Autodesk Inventor part; units mm, degrees
(part 3 of 3)
  spline S581 degree 2 poles (9.4337, -3.0832) (9.3792, -3.0832) (9.2544, -3.1501) (9.1886, -3.2137) knots 0 0 0 1 2 2 2
  spline S582 degree 2 poles (9.1886, -3.2137) (9.1898, -3.2296) (9.192, -3.2738) (9.192, -3.3033) knots 0 0 0 1 2 2 2
  line L532 (9.192, -3.3033) -> (9.192, -3.9954)
  line L533 (9.192, -3.9954) -> (9.0151, -3.9954)
  line L534 (9.0151, -3.9954) -> (9.0151, -3.3873)
  spline S583 degree 2 poles (9.0151, -3.3873) (9.0151, -3.3146) (9.0037, -3.191) (8.9856, -3.1569) knots 0 0 0 1 2 2 2
  spline S584 degree 2 poles (8.9856, -3.1569) (8.9674, -3.1195) (8.8982, -3.0832) (8.8381, -3.0832) knots 0 0 0 1 2 2 2
  spline S585 degree 2 poles (8.8381, -3.0832) (8.7813, -3.0832) (8.6554, -3.1547) (8.5964, -3.2103) knots 0 0 0 1 2 2 2
  line L535 (8.5964, -3.2103) -> (8.5964, -3.9954)
  line L536 (8.5964, -3.9954) -> (8.4194, -3.9954)
  line L537 (8.4194, -3.9954) -> (8.4194, -2.9448)
  line L538 (8.4194, -2.9448) -> (8.5964, -2.9448)
  line L539 (8.5964, -2.9448) -> (8.5964, -3.0605)
  spline S586 degree 2 poles (8.5964, -3.0605) (8.6656, -2.9913) (8.8018, -2.9153) (8.8835, -2.9153) knots 0 0 0 1 2 2 2
  spline S587 degree 2 poles (8.8835, -2.9153) (8.9765, -2.9153) (9.1206, -3.0004) (9.158, -3.0968) knots 0 0 0 1 2 2 2
  spline S588 degree 2 poles (9.158, -3.0968) (9.2386, -3.0072) (9.3906, -2.9153) (9.4791, -2.9153) knots 0 0 0 1 2 2 2
  spline S589 degree 2 poles (9.4791, -2.9153) (9.5471, -2.9153) (9.6583, -2.9573) (9.6992, -3.0049) knots 0 0 0 1 2 2 2
  spline S590 degree 2 poles (9.6992, -3.0049) (9.7412, -3.0526) (9.7877, -3.1955) (9.7877, -3.3033) knots 0 0 0 1 2 2 2
  line L540 (9.7877, -3.3033) -> (9.7877, -3.9954)
  line L541 (9.7877, -3.9954) -> (9.6107, -3.9954)
  line L542 (11.6188, -2.5954) -> (11.2671, -3.9954)
  line L543 (11.2671, -3.9954) -> (11.0583, -3.9954)
  line L544 (11.0583, -3.9954) -> (10.7736, -2.8336)
  line L545 (10.7736, -2.8336) -> (10.4967, -3.9954)
  line L546 (10.4967, -3.9954) -> (10.2903, -3.9954)
  line L547 (10.2903, -3.9954) -> (9.9329, -2.5954)
  line L548 (9.9329, -2.5954) -> (10.1246, -2.5954)
  line L549 (10.1246, -2.5954) -> (10.406, -3.756)
  line L550 (10.406, -3.756) -> (10.6851, -2.5954)
  line L551 (10.6851, -2.5954) -> (10.8745, -2.5954)
  line L552 (10.8745, -2.5954) -> (11.1559, -3.7696)
  line L553 (11.1559, -3.7696) -> (11.4361, -2.5954)
  line L554 (11.4361, -2.5954) -> (11.6188, -2.5954)
  point P0 (0, 0)
  point P1 (17.127, 0)
  constraints: 1 midpoint, 1 point on line, 2 other
extrude "Extrusion3" cut sketch "Sketch3" against normal blind 0.1 contours S211 S212 L234 L235 S213 S214 L5 | L5 S214 S215 S216 S222 S223 S224 S218 S219 S220 S207 S208 S209 S210 S211 | L5 S220 S221 S222 S216 S217 S206 S207 | S0 S1 L10 L11 L12 S2 S3 | L16 L17 L18 L19 L20 L21 | L22 L23 L24 L25 L26 L27 L28 L29 | L30 L31 S8 S9 S10 L32 L33 L34 L35 L36 S11 S12 L37 | S13 S14 S15 S16 | L38 S21 S22 L39 L40 L41 L42 L43 S23 S24 L44 | L45 L46 L47 L48 L49 L50 | S25 S26 S27 S28 S29 S30 L51 S31 S32 S33 L52 L53 S34 S35 S36 L54 L55 L56 | S41 S42 L58 L59 L60 L61 L62 S43 S44 | S49 L64 L65 S50 S51 S52 S53 S54 S55 S56 S57 S58 L66 L67 S59 S60 S61 S62 S63 S64 S65 | L68 L69 L70 L71 L72 L73 | S66 S67 L74 L75 L76 L77 L78 S68 S69 | L82 L83 L84 L85 L86 L87 L88 L89 L90 L91 L92 L93 L94 | L95 L96 L97 L98 | S74 S75 S76 S77 S78 S79 S80 L99 L100 S81 S82 S83 S84 S85 | S93 S94 L101 L102 S95 S96 S97 S98 L103 S99 S100 S101 S102 S103 L104 L105 S104 S105 S106 S107 S108 L106 L107 L108 S109 S110 S111 | S112 S113 S114 L109 L110 S115 S116 S117 S118 S119 S120 S121 L111 L112 L113 L114 L115 S122 S123 S124 | L116 L117 L118 L119 | S125 L120 L121 S126 S127 S128 S129 S130 S131 S132 S133 L122 L123 S134 S135 S136 S137 S138 S139 S140 | L124 L125 L126 L127 L128 L129 L130 L131 L132 L133 L134 L135 L136 | L137 L138 L139 L140 L141 L142 L143 L144 | S141 L148 L149 S142 S143 S144 S145 S146 S147 S148 S149 L150 L151 S150 S151 S152 S153 S154 S155 S156 | L152 L153 L154 L155 | L156 L157 L158 L159 L160 L161 L162 L163 L164 L165 | L166 L167 L168 L169 | L170 L171 L172 L173 | L174 L175 L176 L177 L178 L179 S157 L180 L181 L182 L183 | S158 S159 S160 S161 S162 S163 S164 L184 L185 S165 S166 S167 S168 S169 | L186 L187 L188 L189 L190 L191 S177 L192 L193 L194 L195 | L196 L197 L198 L199 L200 L201 S178 L202 L203 L204 L205 | L206 L207 L208 L209 L210 L211 S179 L212 L213 L214 L215 | S180 S181 S182 L216 L217 S183 S184 S185 S186 S187 S188 S189 L218 L219 L220 L221 L222 S190 S191 S192 | L223 L224 L225 L226 | S193 S194 S195 L227 L228 S196 S197 S198 S199 S200 S201 S202 L229 L230 L231 L232 L233 S203 S204 S205 | S225 S226 S227 S228 S229 S230 L236 L237 S231 S232 S233 S234 S235 S236 S237 S238 L238 L239 S239 S240 | S241 S242 S243 S244 L240 L241 S245 S246 S247 L242 L243 S248 S249 | L245 L246 S254 S255 S256 L247 L248 L249 L250 L251 S257 S258 L252 | S259 L253 L254 L255 L256 L257 L258 L259 L260 L261 L262 L263 S260 S261 S262 L264 L265 S263 | S264 S265 S266 S267 L266 L267 S268 S269 S270 L268 L269 S271 S272 | L271 S277 S278 L272 L273 L274 L275 L276 S279 S280 L277 | L278 L279 L280 L281 L282 L283 L284 L285 L286 L287 L288 L289 L290 | S281 S282 S283 S284 S285 S286 L291 S287 S288 S289 L292 L293 S290 S291 S292 L294 L295 L296 | L298 L299 L300 L301 L302 L303 L304 | S297 S298 S299 S300 L305 L306 S301 S302 S303 L307 L308 S304 S305 | L310 L311 L312 L313 | S310 S311 S312 S313 L314 L315 S314 S315 S316 L316 L317 S317 S318 | L319 L320 S323 S324 S325 L321 L322 L323 L324 L325 S326 S327 L326 | S328 S329 S330 S331 L327 S332 S333 S334 S335 S336 L328 L329 L330 S337 S338 L331 L332 | S343 L334 L335 L336 L337 L338 L339 L340 L341 L342 L343 L344 S344 S345 S346 L345 L346 S347 | L347 L348 S348 S349 S350 L349 L350 L351 L352 L353 S351 S352 L354 | L355 L356 L357 L358 | L359 L360 L361 L362 | S353 S354 S355 S356 S357 S358 S359 L363 L364 S360 S361 S362 S363 S364 | S372 S373 L365 L366 S374 S375 S376 S377 L367 S378 S379 S380 S381 S382 L368 L369 S383 S384 S385 S386 S387 L370 L371 L372 S388 S389 S390 | S391 S392 S393 S394 S395 S396 S397 L373 L374 S398 S399 S400 S401 S402 | L375 L376 L377 L378 | S410 S411 S412 S413 S414 S415 S416 L379 L380 S417 S418 S419 S420 S421 | L381 L382 S429 S430 S431 L383 L384 L385 L386 L387 S432 S433 L388 | L389 S434 S435 S436 S437 L390 L391 L392 S438 S439 S440 L393 L394 L395 L396 L397 S441 S442 S443 S444 S445 L398 L399 | L400 L401 L402 L403 L404 L405 L406 L407 L408 L409 | L410 L411 L412 L413 | L414 L415 L416 L417 | S446 S447 L418 L419 L420 L421 L422 S448 S449 | S454 S455 S456 S457 L424 L425 S458 S459 S460 L426 L427 S461 S462 | L429 S467 S468 L430 L431 L432 L433 L434 S469 S470 L435 | S471 S472 S473 S474 S475 S476 S477 S478 | L436 L437 S485 S486 S487 L438 L439 L440 S488 S489 S490 L441 L442 L443 | S491 L444 L445 L446 L447 L448 L449 L450 L451 L452 L453 L454 S492 S493 S494 L455 L456 S495 | S496 S497 L457 L458 L459 L460 L461 S498 S499 | L463 L464 S504 S505 S506 L465 L466 L467 S507 S508 S509 L468 L469 L470 | S510 L471 L472 L473 L474 L475 L476 L477 L478 L479 L480 L481 S511 S512 S513 L482 L483 S514 | S515 S516 L484 L485 L486 L487 L488 S517 S518 | S523 S524 S525 S526 | L492 L493 L494 L495 L496 L497 L498 L499 L500 L501 L502 L503 L504 | S531 S532 S533 S534 L505 L506 S535 S536 S537 L507 L508 S538 S539 | L510 S544 S545 L511 L512 L513 L514 L515 S546 S547 L516 | L517 L518 L519 L520 | L521 L522 L523 L524 | S548 S549 S550 L525 S551 S552 S553 S554 L526 S555 S556 | L527 L528 L529 L530 | S567 S568 S569 S570 | L531 S579 S580 S581 S582 L532 L533 L534 S583 S584 S585 L535 L536 L537 L538 L539 S586 S587 S588 S589 S590 L540 L541 | L542 L543 L544 L545 L546 L547 L548 L549 L550 L551 L552 L553 L554
body "Solid1"
